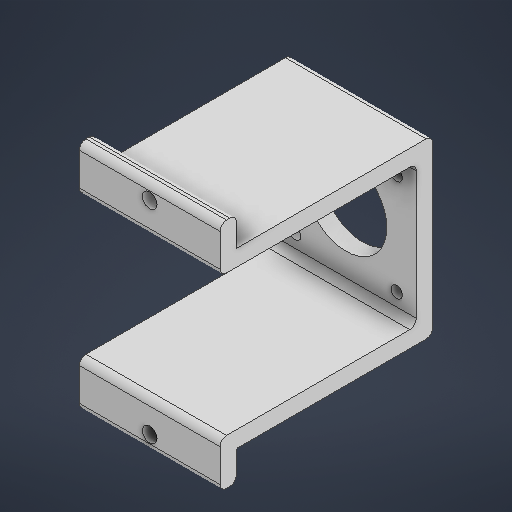
# Autodesk Inventor part: motor_holder_V4
Saved by Autodesk Inventor 2026 (Build 300175050, 175E)
## iProperties
Created: 2025-09-11
Part Number: motor_holder_V4
Material: Generic
Document SubType Name: Modeling
Designer: aduwa
Density: 1 g/cm^3
Appearance: Default
Author: aduwa
Autodesk Inventor part; units mm, degrees
ref_plane "YZ Plane" through (0, 0, 0) normal (1, 0, 0) x (0, 1, 0)
ref_plane "XZ Plane" through (0, 0, 0) normal (0, 1, 0) x (-1, 0, 0)
ref_plane "XY Plane" through (0, 0, 0) normal (0, 0, 1) x (1, 0, 0)
sketch "Sketch1" plane through (0, 0, 0) normal (0, 0, 1) x (1, 0, 0)
  circle A0 centre (-15.5, -15.5) radius 1.75
  circle A1 centre (15.5, -15.5) radius 1.75
  circle A2 centre (-15.5, 15.5) radius 1.75
  circle A3 centre (15.5, 15.5) radius 1.75
  circle A4 centre (0, 0) radius 12.5
  line L0 (-21.5, 21.5) -> (21.5, 21.5)
  line L1 (21.5, -21.5) -> (-21.5, -21.5)
  line L2 (-21.5, 21.5) -> (21.5, -21.5) construction
  line L3 (21.5, 21.5) -> (-21.5, -21.5) construction
  line L4 (-21.5, -21.5) -> (21.5, -21.5)
  line L5 (-21.5, 21.5) -> (-21.5, -21.5)
  line L6 (21.5, 21.5) -> (21.5, -21.5)
  line L7 (-21.5, 21.5) -> (21.5, 21.5)
  line L8 (21.5, 21.5) -> (21.5, 26.5)
  line L9 (21.5, 26.5) -> (-21.5, 26.5)
  line L10 (-21.5, 26.5) -> (-21.5, 21.5)
  line L11 (0, 0) -> (-7.0913, 0)
  line L12 (21.5, -21.5) -> (21.5, -26.5)
  line L13 (21.5, -26.5) -> (-21.5, -26.5)
  line L14 (-21.5, -26.5) -> (-21.5, -21.5)
  point P0 (0, 26.5)
  point P1 (0, -26.5)
  point P2 (21.5, 21.5)
  dimension "d0" = 3.5
  dimension "d1" = 31
  dimension "d2" = 25
  dimension "d3" = 43
  dimension "d4" = 43
  dimension "d6" = 15.5
  dimension "d7" = 43
  dimension "d8" = 5
  constraints: 30 end point, 5 centre point, 5 symmetric about line, 4 horizontal, 3 equal radius, 3 midpoint, 3 parallel, 3 point on line, 3 vertical alignment, 1 coincident, 1 horizontal alignment, 1 perpendicular, 1 vertical
  measures "d0" diameter of A0
  measures "d1" distance of A0.centre A2.centre
  measures "d2" diameter of A4
  measures "d3" distance of L2.end L3.end
  measures "d4" distance of L3.start L2.end
  measures "d6" horizontal distance of L11.start A2.centre
  measures "d7" distance of L9.end L8.end
  measures "d8" distance of L8.end L7.end
extrude "face" add sketch "Sketch1" against normal blind 5
extrude "length" add sketch "Sketch1" along normal blind 55 contours L10 L9 L8 L0 | L1 L12 L13 L14
sketch "Sketch2" plane through (0, 0, 55) normal (0, 0, 1) x (1, 0, 0)
  line L0 (-21.5, -21.5) -> (21.5, -21.5) projected
  line L1 (21.5, -21.5) -> (21.5, 21.5) projected
  line L2 (21.5, 21.5) -> (-21.5, 21.5) projected
  line L3 (-21.5, 21.5) -> (-21.5, -21.5) projected
  circle A0 centre (15.5, 15.5) radius 1.75 projected
  circle A1 centre (-15.5, 15.5) radius 1.75 projected
  circle A2 centre (-15.5, -15.5) radius 1.75 projected
  circle A3 centre (15.5, -15.5) radius 1.75 projected
  circle A4 centre (0, 0) radius 12.5 projected
  line L4 (-21.5, 26.5) -> (-21.5, 21.5) projected
  line L5 (-21.5, 21.5) -> (21.5, 21.5) projected
  line L6 (21.5, 21.5) -> (21.5, 26.5) projected
  line L7 (21.5, 26.5) -> (-21.5, 26.5) projected
  line L8 (21.5, -26.5) -> (21.5, -21.5) projected
  line L9 (21.5, -21.5) -> (-21.5, -21.5) projected
  line L10 (-21.5, -21.5) -> (-21.5, -26.5) projected
  line L11 (-21.5, -26.5) -> (21.5, -26.5) projected
  line L12 (-21.5, 26.5) -> (21.5, 26.5)
  line L13 (21.5, 26.5) -> (21.5, 35.5)
  line L14 (21.5, 35.5) -> (-21.5, 35.5)
  line L15 (-21.5, 35.5) -> (-21.5, 26.5)
  line L16 (0, 0) -> (-5.3455, 0)
  line L17 (21.5, -26.5) -> (21.5, -35.5)
  line L18 (21.5, -35.5) -> (-21.5, -35.5)
  line L19 (-21.5, -35.5) -> (-21.5, -26.5)
  line L20 (-21.5, -26.5) -> (21.5, -26.5) projected
  circle A5 centre (0, -31) radius 2.25
  circle A6 centre (0, 31) radius 2.25
  point P0 (-21.5, -31)
  dimension "d13" = 9
  dimension "d19" = 4.5
  constraints: 16 end point, 4 symmetric about line, 3 parallel, 2 centre point, 2 horizontal, 1 horizontal alignment, 1 midpoint, 1 perpendicular, 1 other
  measures "d13" distance of L13.end L12.end
  measures "d19" diameter of A5
extrude "mount" add sketch "Sketch2" along normal blind 5 contours L0 L8 L11 L10 | L4 L7 L6 L2 | L11 L17 L18 L19 | L15 L14 L13 L7
fillet "Fillet3" radius 2 2 edges at (0, -21.5, 0) (0, 21.5, 0)
fillet "Fillet4" radius 2 2 edges at (0, 21.5, 60) (0, -21.5, 60)
fillet "Fillet5" radius 2 6 edges at (0, -26.5, -5) (0, 26.5, -5) (0, 35.5, 55) (0, 35.5, 60) (0, -35.5, 55) (0, -35.5, 60)
body "Solid1"
